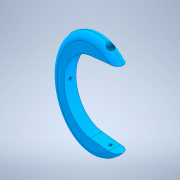
# Autodesk Inventor part: BodyDampener V2
Saved by Autodesk Inventor 2022.2 (Build 262287030, 287C)
## iProperties
Created: 2022-03-24
Part Number: BodyDampener V2
Material: Generic
Document SubType Name: Modeling
Designer: Jochen
Density: 1 g/cm^3
Appearance: Default
Author: Jochen
Autodesk Inventor part; units mm, degrees
ref_plane "YZ Plane" through (0, 0, 0) normal (1, 0, 0) x (0, 1, 0)
ref_plane "XZ Plane" through (0, 0, 0) normal (0, 1, 0) x (-1, 0, 0)
ref_plane "XY Plane" through (0, 0, 0) normal (0, 0, 1) x (1, 0, 0)
sketch "Sketch1" plane through (0, 0, 0) normal (0, 0, 1) x (1, 0, 0)
  line L0 (0, 28.4285) -> (0, -28.4285) construction
  line L1 (0, 28.4285) -> (-43.0257, 28.4285) construction
  line L2 (-43.0257, -28.4285) -> (-43.0257, 28.4285) construction
  line L3 (0, -28.4285) -> (-43.0257, -28.4285) construction
  line L4 (-29, -28.4285) -> (-29, 28.4285) construction
  line L5 (0, 28.4285) -> (-29, 28.4285) construction
  line L6 (0, 28.4285) -> (-9, 27.4285)
  ellipse E0 centre (-7.0663, 0) end of major axis (-7.0663, -27.5357) minor radius 21.9337 (-9, 27.4285) -> (-9, -27.4285) ccw
  line L7 (0, 28.4285) -> (0, -28.4285) construction
  line L8 (0, 28.4285) -> (0, -28.4285)
  line L9 (0, -28.4285) -> (-29, -28.4285) construction
  line L10 (0, -28.4285) -> (-29, -28.4285)
  line L11 (0, -28.4285) -> (-29, -28.4285)
  line L12 (0, -28.4285) -> (-9, -27.4285)
  line L13 (0, 0.1054) -> (0, 0.565) construction
  line L14 (0, -28.4285) -> (18, -30.4285) construction
  line L15 (18, -30.4285) -> (18, -28.4285) construction
  line L16 (-43.0257, 28.4285) -> (-43.0257, -28.4285) construction
  line L17 (-43.0257, 0) -> (0, 0) construction
  line L18 (0, -28.4285) -> (0, 28.4285) construction
  line L19 (-9, -27.4285) -> (-9, 27.4285) construction
  line L20 (0, -59.2648) -> (0, 75.5888) construction
  line L21 (-76.2, 0) -> (37.2, 0) construction
  line L22 (0, 28.4285) -> (5, 28.9841)
  line L23 (0, -28.4285) -> (10, -29.5396)
  line L24 (5, 28.9841) -> (11.675, 28.9841)
  line L25 (5, -28.9841) -> (11.675, -28.9841)
  line L26 (10.2027, -28.9841) -> (10.2027, -29.5621)
  ellipse E1 centre (-9, 0) end of major axis (-9.0655, 25.1712) minor radius 20 construction
  ellipse E2 centre (-9, 0) end of major axis (-9, 40) minor radius 30
  point P0 (-60, 28.4445)
  point P1 (-13, 43)
  point P2 (-13, 56.324)
  point P3 (-13, 11)
  point P4 (-13, 0.565)
  point P5 (0, 0.3352)
  point P6 (-9, 0)
  point P7 (-39, 0)
  point P8 (-29, 0)
  point P9 (-9, 40)
  point P10 (-9, -40)
  dimension "d0" = 2
  dimension "d1" = 18
  dimension "d2" = 29
  dimension "d3" = 9
  dimension "d4" = 20
  dimension "d5" = 56.857
  dimension "d8" = 5
  dimension "d31" = 5
  dimension "d34" = 10
  dimension "d35" = 40
  constraints: 51 end point, 8 midpoint, 6 point on line, 3 coincident, 3 perpendicular, 3 vertical, 2 collinear, 2 horizontal, 1 horizontal alignment, 1 symmetric about line, 21 other
  measures "d0" distance of L14.end L15.end
  measures "d1" distance from line of L0.end L15
  measures "d2" distance between parallel lines of L0 L4
  measures "d3" distance between parallel lines of L0 L19
  measures "d4" distance between parallel lines of L19 L4
  measures "d5" distance of L2.start L1.end
  measures "d8" distance from line of L0 L22.end
  measures "d31" distance from line of L25.start L0
  measures "d34" distance of point (-29, 0) point (-39, 0)
  measures "d35" distance from line of L17 point (-9, 40)
extrude "Extrusion1" add sketch "Sketch1" along normal blind 9 contours L6 E0 L12 L23 L25 E2 L24 L22
fillet "Fillet1" radius 4.5 2 edges at (-39, 0, 9) (-39, 0, 0)
sketch "Sketch2" plane through (0, 0, 0) normal (0, 1, 0) x (-1, 0, 0)
  line L0 (0, -1.8) -> (0, 10.8) construction
  line L1 (1.6, 0) -> (-6.1, 0) construction
  circle A0 centre (-2, 4.5) radius 1
  line L2 (-5, 0) -> (-5, 9) projected
  circle A1 centre (-2, 4.5) radius 2.5
  point P0 (0, 0)
  dimension "d13" = 2
  dimension "d14" = 3
  dimension "d15" = 4.5
  dimension "d18" = 5
  constraints: 2 centre point, 1 coincident
  measures "d13" diameter of A0
  measures "d14" distance from line of A0.centre L2
  measures "d15" distance from line of L1 A0.centre
  measures "d18" diameter of A1
extrude "Extrusion3" add sketch "Sketch2" along normal through all both and the other way through all separate body contours A0 | A1
extrude "Extrusion4" cut sketch "Sketch2" along normal mid plane 68 contours A0 | A1 bodies 2
combine bodies "Combine1" operation type subtract main body 1 bodies to subtract 2
extrude "Extrusion2" cut sketch "Sketch2" along normal through all both and the other way through all contours A0 bodies 1
sketch "Sketch3" plane through (0, 0, 0) normal (1, 0, 0) x (0, 1, 0)
  line L0 (37.3673, 4.5) -> (-37.3673, 4.5) construction
  circle A0 centre (0, 4.5) radius 1
  circle A1 centre (0, 4.5) radius 2.5
  point P0 (0, 0)
  dimension "d23" = 2
  dimension "d24" = 5
  constraints: 2 centre point, 1 coincident, 1 midpoint
  measures "d23" diameter of A0
  measures "d24" diameter of A1
extrude "Extrusion8" cut sketch "Sketch3" against normal blind 50 contours A0 bodies 1
extrude "Extrusion6" add sketch "Sketch3" against normal blind 40 separate body contours A0
extrude "Extrusion7" cut sketch "Sketch3" along normal blind 6 from surface at -40 contours A0 | A1 bodies 1
body "Solid4"
